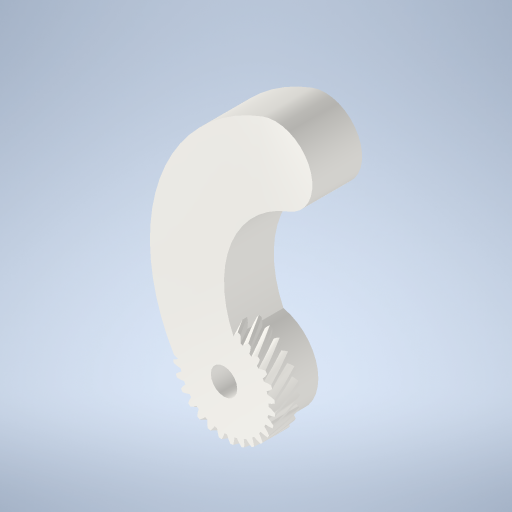
# Autodesk Inventor part: Spur Gear1
Saved by Autodesk Inventor 2024 (Build 280153000, 153)
## iProperties
CustomPartVersion: 1
Created: 2023-09-14
Part Number: Spur Gear1
Material: Steel
Document SubType Name: Modeling
Designer: jebes windows
Categories: <?xml version="1.0" encoding="UTF-16"?> <MemberInstance><Categories><FamilyTemplate><FamilyTemplateParameter ValueType="xs:double" Id="1" ObjectReferenceKey="da_z" ObjectType="kUserParameterObject"/><FamilyTemplateParameter ValueType="xs:double" Id="2" ObjectReferenceKey="da_b" ObjectType="kUserParameterObject"/><FamilyTemplateParameter ValueType="xs:double" Id="3" ObjectReferenceKey="da_beta" ObjectType="kUserParameterObject"/><FamilyTemplateParameter ValueType="xs:double" Id="4" ObjectReferenceKey="da_da" ObjectType="kUserParameterObject"/><FamilyTemplateParameter ValueType="xs:double" Id="5" ObjectReferenceKey="da_aw" ObjectType="kUserParameterObject"/><FamilyTemplateParameter ValueType="xs:string" Id="6" ObjectReferenceKey="EAIAABAAAACIAQAAAAAAAIAAAAAAAAAA" ObjectType="83910656" SubObjectId="SurfaceGeometry"/></FamilyTemplate><ParamToTemplateMap><ParamToTemplate CategoryParameter="//CategoryParameter[@InternalName='046C89C9-8512-4d59-83FE-43B91F4F132A']" TemplateParameter="1"/><ParamToTemplate CategoryParameter="//CategoryParameter[@InternalName='2552DF32-E462-4b46-AEBF-C6C7768E72AC']" TemplateParameter="2"/><ParamToTemplate CategoryParameter="//CategoryParameter[@InternalName='C9EE641D-15FC-4fae-A226-E94C4372FDD7']" TemplateParameter="3"/><ParamToTemplate><ParamToTemplate CategoryParameter="//CategoryParameter[@InternalName='00B6519A-459B-49c7-AD84-2E56D39A5744']" ConstantValue="0.000000"/></ParamToTemplate><ParamToTemplate><ParamToTemplate CategoryParameter="//CategoryParameter[@InternalName='04B31F0E-C7A6-4894-AA32-9629BEFACF47']" ConstantValue="1.000000"/></ParamToTemplate><ParamToTemplate><ParamToTemplate CategoryParameter="//CategoryParameter[@InternalName='43CBEC2E-7847-49e7-A936-2F7889FCB2D9']" ConstantValue="0.250000"/></ParamToTemplate><ParamToTemplate><ParamToTemplate CategoryParameter="//CategoryParameter[@InternalName='B1EFC894-105D-4ebd-86BF-FA20ED196853']" ConstantValue="0.302500"/></ParamToTemplate><ParamToTemplate><ParamToTemplate CategoryParameter="//CategoryParameter[@InternalName='51175063-3D10-4879-93E8-6246FE8B403D']" ConstantValue="2060000000.000000"/></ParamToTemplate><ParamToTemplate><ParamToTemplate CategoryParameter="//CategoryParameter[@InternalName='A3A52E27-4454-46a9-B0BD-C932399B70AF']" ConstantValue="0.300000"/></ParamToTemplate><ParamToTemplate><ParamToTemplate CategoryParameter="//CategoryParameter[@InternalName='91B76062-C214-41d9-B1B9-14D2AB99603D']" ConstantValue="0.060000"/></ParamToTemplate><ParamToTemplate><ParamToTemplate CategoryParameter="//CategoryParameter[@InternalName='374E806E-8B8A-4dda-A9AA-1039D6500AD2']" ConstantValue="16.666667"/></ParamToTemplate><ParamToTemplate><ParamToTemplate CategoryParameter="//CategoryParameter[@InternalName='2D373A89-B862-43d6-8D0B-0CBF12AB9F6C']" ConstantValue="0.436332"/></ParamToTemplate><ParamToTemplate CategoryParameter="//CategoryParameter[@InternalName='37777632-D6A2-4fac-9D53-DB8ACD95C989']" TemplateParameter="4"/><ParamToTemplate CategoryParameter="//CategoryParameter[@InternalName='FD1017F1-B727-4f7e-9707-0F86F1FF9423']" TemplateParameter="5"/><ParamToTemplate><ParamToTemplate CategoryParameter="//CategoryParameter[@InternalName='9E1B4470-B2D3-4ff1-B813-535BB4CDF51A']" ConstantValue="3520000.000000"/></ParamToTemplate><ParamToTemplate><ParamToTemplate CategoryParameter="//CategoryParameter[@InternalName='F8452263-BFF6-458c-9FB1-07C4B99E95CD']" ConstantValue="11400000.000000"/></ParamToTemplate><ParamToTemplate><ParamToTemplate CategoryParameter="//CategoryParameter[@InternalName='3E3BB259-FD49-497f-8171-6EBC954A3479']" ConstantValue="2.000000"/></ParamToTemplate><ParamToTemplate CategoryParameter="//CategoryParameter[@InternalName='27C3BAF2-7550-4e4b-AE2C-0DB134B7D9B7']" TemplateParameter="6"/></ParamToTemplateMap><Category DisplayName="Gear" InternalName="DC85795E-93AB-48d5-8EEE-5A27447B64BD" Mnemonic="Gear"><CategoryParameter DisplayName="z" InternalName="046C89C9-8512-4d59-83FE-43B91F4F132A" Mnemonic="z"/><CategoryParameter DisplayName="b" InternalName="2552DF32-E462-4b46-AEBF-C6C7768E72AC" Mnemonic="b"/><CategoryParameter DisplayName="||b|" InternalName="C9EE641D-15FC-4fae-A226-E94C4372FDD7" Mnemonic="beta"/><CategoryParameter DisplayName="x" InternalName="00B6519A-459B-49c7-AD84-2E56D39A5744" Mnemonic="x"/><CategoryParameter DisplayName="a*" InternalName="04B31F0E-C7A6-4894-AA32-9629BEFACF47" Mnemonic="a"/><CategoryParameter DisplayName="c*" InternalName="43CBEC2E-7847-49e7-A936-2F7889FCB2D9" Mnemonic="c"/><CategoryParameter DisplayName="r|.f|*" InternalName="B1EFC894-105D-4ebd-86BF-FA20ED196853" Mnemonic="rf"/><CategoryParameter DisplayName="E" InternalName="51175063-3D10-4879-93E8-6246FE8B403D" Mnemonic="E"/><CategoryParameter DisplayName="||m|" InternalName="A3A52E27-4454-46a9-B0BD-C932399B70AF" Mnemonic="mi"/><Category DisplayName="SpurGear" InternalName="26C5A22E-A91E-4dfd-A3B3-23CCAFAE1764" Mnemonic="SpurGear"><CategoryParameter DisplayName="m" InternalName="91B76062-C214-41d9-B1B9-14D2AB99603D" Mnemonic="m"/><CategoryParameter DisplayName="P" InternalName="374E806E-8B8A-4dda-A9AA-1039D6500AD2" Mnemonic="PP"/><CategoryParameter DisplayName="||a|" InternalName="2D373A89-B862-43d6-8D0B-0CBF12AB9F6C" Mnemonic="alpha"/><CategoryParameter DisplayName="d|.a|" InternalName="37777632-D6A2-4fac-9D53-DB8ACD95C989" Mnemonic="da"/><CategoryParameter DisplayName="a|.w|" InternalName="FD1017F1-B727-4f7e-9707-0F86F1FF9423" Mnemonic="aw"/><CategoryParameter DisplayName="||s||.Flim|" InternalName="9E1B4470-B2D3-4ff1-B813-535BB4CDF51A" Mnemonic="sFlim"/><CategoryParameter DisplayName="||s||.Hlim|" InternalName="F8452263-BFF6-458c-9FB1-07C4B99E95CD" Mnemonic="sHlim"/><CategoryParameter DisplayName="type" InternalName="3E3BB259-FD49-497f-8171-6EBC954A3479" Mnemonic="type"/><CategoryParameter DisplayName="PitchDiameter" InternalName="27C3BAF2-7550-4e4b-AE2C-0DB134B7D9B7" Mnemonic="IDS_PITCHDIAM"/></Category></Category></Categories></MemberInstance>
Density: 1 g/cm^3
Appearance: Steel
Author: jebes windows
## iProperties of the stored document Spur Gear12_3DPrint.ipt
Created: 2023-09-14
Part Number: Spur Gear12_3DPrint
Material: Generic
Document SubType Name: Modeling
Designer: jebes windows
Density: 1 g/cm^3
Appearance: Default
Author: jebes windows
Autodesk Inventor part; units mm, degrees
sketch "Sketch1" plane through (0, 0, 0) normal (0, 0, 1) x (1, 0, 0)
  circle A0 centre (0, 0) radius 10.294
  dimension "d0" = 20.5879
  constraints: 1 centre point
  measures "d0" diameter of A0
extrude "Extrusion1" add sketch "Sketch1" along normal blind 5
ref_plane "Work Plane2" through (0, 0, 2.5) normal (0, 0, 1) x (1, 0, 0)
sketch "Sketch2" plane through (0, 0, 0) normal (0, 0, -1) x (-1, 0, 0)
  circle A0 centre (0, 0) radius 10.294 projected
  circle A1 centre (0, 0) radius 9.6995
  dimension "d3" = 19.399
  constraints: 1 centre point, 1 coincident
  measures "d3" diameter of A1
surface extrude "Pitch Diameter" sketch "Sketch2" against normal through all shown no curves A1
ref_plane "Work Plane8" through (0, 0, 0) normal (0.9937122, 0.1119645, 0) x (0, 0, 1)
ref_plane "Work Plane9" through (0, 0, 0) normal (1, 0, 0) x (0, 1, 0)
spur gear teeth "Spur Gear" teeth 28 pitch diameter 19.399 tip diameter 20.5879 root diameter 17.899 face width 5 helix angle 30 hand left start plane through (0, 0, 0) normal (0, 0, -1) x (-1, 0, 0)
sketch "Sketch3" plane through (0, 0, 0) normal (0, 0, -1) x (-1, 0, 0)
  circle A0 centre (0, 0) radius 2.65
  dimension "d49" = 5.3
  constraints: 1 centre point, 1 coincident
  measures "d49" diameter of A0
extrude "Extrusion2" cut sketch "Sketch3" against normal blind 10
sketch "Sketch4" plane through (0, 0, 0) normal (0, 0, -1) x (-1, 0, 0)
  line L0 (0, 0) -> (10, 0)
  line L1 (0, 0) -> (-10, 0)
  circle A0 centre (-20, 17.3205) radius 20
  circle A1 centre (0, 0) radius 2.65 projected
  arc A2 (2.5712, 9.9677) -> (2.0083, 10.0962) centre (0, 0) ccw projected
  arc A3 (0.2887, 10.2899) -> (-0.2887, 10.2899) centre (0, 0) ccw projected
  arc A4 (-2.0083, 10.0962) -> (-2.5712, 9.9677) centre (0, 0) ccw projected
  spline S0 degree 5 poles (-2.7178, 8.5268) (-2.8134, 8.4964) (-2.9087, 8.4645) (-3.0035, 8.4313) (-3.0978, 8.3969) (-3.1916, 8.361) knots 0 0 0 0 0 0 1 1 1 1 1 1 projected
  arc A5 (-4.2045, 9.3962) -> (-4.7247, 9.1456) centre (0, 0) ccw projected
  spline S1 degree 5 poles (-4.547, 7.7083) (-4.6335, 7.6573) (-4.7193, 7.6051) (-4.8043, 7.5516) (-4.8886, 7.497) (-4.9721, 7.4412) knots 0 0 0 0 0 0 1 1 1 1 1 1 projected
  arc A6 (-6.1899, 8.225) -> (-6.6414, 7.865) centre (0, 0) ccw projected
  spline S2 degree 5 poles (-6.1483, 6.5032) (-6.2212, 6.4343) (-6.2932, 6.3642) (-6.3642, 6.2932) (-6.4343, 6.2212) (-6.5032, 6.1483) knots 0 0 0 0 0 0 1 1 1 1 1 1 projected
  arc A7 (-7.865, 6.6414) -> (-8.225, 6.1899) centre (0, 0) ccw projected
  spline S3 degree 5 poles (-7.4412, 4.9721) (-7.497, 4.8886) (-7.5516, 4.8043) (-7.6051, 4.7193) (-7.6573, 4.6335) (-7.7083, 4.547) knots 0 0 0 0 0 0 1 1 1 1 1 1 projected
  arc A8 (-9.1456, 4.7247) -> (-9.3962, 4.2045) centre (0, 0) ccw projected
  spline S4 degree 5 poles (-8.361, 3.1916) (-8.3969, 3.0978) (-8.4313, 3.0035) (-8.4645, 2.9087) (-8.4964, 2.8134) (-8.5268, 2.7178) knots 0 0 0 0 0 0 1 1 1 1 1 1 projected
  arc A9 (-9.9677, 2.5712) -> (-10.0962, 2.0083) centre (0, 0) ccw projected
  spline S5 degree 5 poles (-8.8616, 1.2511) (-8.8756, 1.1516) (-8.8883, 1.052) (-8.8995, 0.9522) (-8.9094, 0.8523) (-8.9178, 0.7522) knots 0 0 0 0 0 0 1 1 1 1 1 1 projected
  arc A10 (-10.2899, 0.2887) -> (-10.2899, -0.2887) centre (0, 0) ccw projected
  spline S6 degree 5 poles (-8.9178, -0.7522) (-8.9094, -0.8523) (-8.8995, -0.9522) (-8.8883, -1.052) (-8.8756, -1.1516) (-8.8616, -1.2511) knots 0 0 0 0 0 0 1 1 1 1 1 1 projected
  arc A11 (-10.0962, -2.0083) -> (-9.9677, -2.5712) centre (0, 0) ccw projected
  spline S7 degree 5 poles (-8.5268, -2.7178) (-8.4964, -2.8134) (-8.4645, -2.9087) (-8.4313, -3.0035) (-8.3969, -3.0978) (-8.361, -3.1916) knots 0 0 0 0 0 0 1 1 1 1 1 1 projected
  arc A12 (-9.3962, -4.2045) -> (-9.1456, -4.7247) centre (0, 0) ccw projected
  spline S8 degree 5 poles (-7.7083, -4.547) (-7.6573, -4.6335) (-7.6051, -4.7193) (-7.5516, -4.8043) (-7.497, -4.8886) (-7.4412, -4.9721) knots 0 0 0 0 0 0 1 1 1 1 1 1 projected
  arc A13 (-8.225, -6.1899) -> (-7.865, -6.6414) centre (0, 0) ccw projected
  spline S9 degree 5 poles (-6.5032, -6.1483) (-6.4343, -6.2212) (-6.3642, -6.2932) (-6.2932, -6.3642) (-6.2212, -6.4343) (-6.1483, -6.5032) knots 0 0 0 0 0 0 1 1 1 1 1 1 projected
  arc A14 (-6.6414, -7.865) -> (-6.1899, -8.225) centre (0, 0) ccw projected
  spline S10 degree 5 poles (-4.9721, -7.4412) (-4.8886, -7.497) (-4.8043, -7.5516) (-4.7193, -7.6051) (-4.6335, -7.6573) (-4.547, -7.7083) knots 0 0 0 0 0 0 1 1 1 1 1 1 projected
  arc A15 (-4.7247, -9.1456) -> (-4.2045, -9.3962) centre (0, 0) ccw projected
  spline S11 degree 5 poles (-3.1916, -8.361) (-3.0978, -8.3969) (-3.0035, -8.4313) (-2.9087, -8.4645) (-2.8134, -8.4964) (-2.7178, -8.5268) knots 0 0 0 0 0 0 1 1 1 1 1 1 projected
  arc A16 (-2.5712, -9.9677) -> (-2.0083, -10.0962) centre (0, 0) ccw projected
  spline S12 degree 5 poles (-1.2511, -8.8616) (-1.1516, -8.8756) (-1.052, -8.8883) (-0.9522, -8.8995) (-0.8523, -8.9094) (-0.7522, -8.9178) knots 0 0 0 0 0 0 1 1 1 1 1 1 projected
  arc A17 (-0.2887, -10.2899) -> (0.2887, -10.2899) centre (0, 0) ccw projected
  spline S13 degree 5 poles (0.7522, -8.9178) (0.8523, -8.9094) (0.9522, -8.8995) (1.052, -8.8883) (1.1516, -8.8756) (1.2511, -8.8616) knots 0 0 0 0 0 0 1 1 1 1 1 1 projected
  arc A18 (2.0083, -10.0962) -> (2.5712, -9.9677) centre (0, 0) ccw projected
  spline S14 degree 5 poles (2.7178, -8.5268) (2.8134, -8.4964) (2.9087, -8.4645) (3.0035, -8.4313) (3.0978, -8.3969) (3.1916, -8.361) knots 0 0 0 0 0 0 1 1 1 1 1 1 projected
  arc A19 (4.2045, -9.3962) -> (4.7247, -9.1456) centre (0, 0) ccw projected
  arc A20 (6.1899, -8.225) -> (6.6414, -7.865) centre (0, 0) ccw projected
  arc A21 (7.865, -6.6414) -> (8.225, -6.1899) centre (0, 0) ccw projected
  arc A22 (9.1456, -4.7247) -> (9.3962, -4.2045) centre (0, 0) ccw projected
  spline S15 degree 5 poles (8.361, -3.1916) (8.3969, -3.0978) (8.4313, -3.0035) (8.4645, -2.9087) (8.4964, -2.8134) (8.5268, -2.7178) knots 0 0 0 0 0 0 1 1 1 1 1 1 projected
  arc A23 (9.9677, -2.5712) -> (10.0962, -2.0083) centre (0, 0) ccw projected
  spline S16 degree 5 poles (8.8616, -1.2511) (8.8756, -1.1516) (8.8883, -1.052) (8.8995, -0.9522) (8.9094, -0.8523) (8.9178, -0.7522) knots 0 0 0 0 0 0 1 1 1 1 1 1 projected
  spline S17 degree 5 poles (8.9178, -0.7522) (9.2027, -0.6957) (9.484, -0.6207) (9.76, -0.5275) (10.0291, -0.4166) (10.2899, -0.2887) knots 0 0 0 0 0 0 1 1 1 1 1 1 projected
  arc A24 (10.2899, -0.2887) -> (10.2899, 0.2887) centre (0, 0) ccw projected
  arc A25 (10.0962, 2.0083) -> (9.9677, 2.5712) centre (0, 0) ccw projected
  arc A26 (9.3962, 4.2045) -> (9.1456, 4.7247) centre (0, 0) ccw projected
  arc A27 (8.225, 6.1899) -> (7.865, 6.6414) centre (0, 0) ccw projected
  arc A28 (6.6414, 7.865) -> (6.1899, 8.225) centre (0, 0) ccw projected
  arc A29 (4.7247, 9.1456) -> (4.2045, 9.3962) centre (0, 0) ccw projected
  circle A30 centre (-20, 17.3205) radius 34.8959
  circle A31 centre (-10.307, 43) radius 7.448
  circle A32 centre (0, 0) radius 8.9495
  point P0 (-2.65, 0)
  point P1 (2.65, 0)
  point P2 (-10.294, 0)
  point P3 (-10.2926, -0.1657)
  point P4 (1.8486, -9.8891)
  point P5 (2.6978, -9.1849)
  point P6 (3.3738, -8.5907)
  point P7 (8.4904, -2.8294)
  point P8 (8.5684, -2.7188)
  point P9 (9.3767, -1.5139)
  point P10 (10.0663, -0.3923)
  point P11 (-7.6768, 49.9681)
  point P12 (-12.9372, 36.0319)
  point P13 (-8.9, -0.9396)
  point P14 (-8.5076, -2.7775)
  point P15 (-7.7083, -4.547)
  point P16 (-7.4412, -4.9721)
  point P17 (-6.3282, -6.3282)
  point P18 (-6.1483, -6.5032)
  point P19 (-4.9721, -7.4412)
  point P20 (-4.547, -7.7083)
  point P21 (-3.1916, -8.361)
  point P22 (-2.7775, -8.5076)
  point P23 (-0.9396, -8.9)
  point P24 (0.9396, -8.9)
  point P25 (2.7775, -8.5076)
  point P26 (4.0133, -7.9992)
  point P27 (8.4904, -2.8294)
  point P28 (8.5076, -2.7775)
  point P29 (8.9, -0.9396)
  point P30 (-1.9352, 8.7377)
  point P31 (-2.7775, 8.5076)
  point P32 (-4.601, 7.6762)
  point P33 (-4.9721, 7.4412)
  point P34 (-6.1483, 6.5032)
  point P35 (-6.5032, 6.1483)
  point P36 (-7.4412, 4.9721)
  point P37 (-7.7083, 4.547)
  point P38 (-8.361, 3.1916)
  point P39 (-8.5076, 2.7775)
  point P40 (-8.8616, 1.2511)
  point P41 (-8.9, 0.9396)
  dimension "d54" = 40
  dimension "d52" = 10
  dimension "d53" = 10
  dimension "d55" = 20
  dimension "d62" = 69.7918
  dimension "d63" = 43
  constraints: 4 end point, 2 centre point, 2 coincident, 2 horizontal, 1 point on circle, 1 tangent, 91 other
  measures "d52" distance of L0.start L0.end
  measures "d53" distance of L0.start L1.end
  measures "d55" horizontal distance of L0.start point (-20, 17.321)
  measures "d62" diameter of A30
  measures "d63" distance of A31.centre point (-10.294, 0)
extrude "Extrusion3" add sketch "Sketch4" along normal mid plane 10 contours A1 L1 A32 A0 L0 | L0 A32 S16 S15 A30 S14 S13 S12 S11 S10 S9 S8 S7 S6 L1 A1 | A32 A0 A31 A30 S17 | A0 A32 S5 S4 S3 S2 S1 S0 | A31 picked at (-5.5744, 4.7783)
equation "\"d0\" = da_da"
equation "\"d1\" = da_b"
equation "\"d3\" = da_d"
equation "\"da_da\" = 20.587946"
equation "\"da_b\" = 5"
equation "\"da_d\" = 19.398969"
body "Solid1"
body "Srf1"
